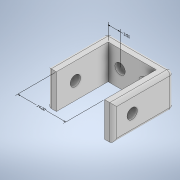
# Autodesk Inventor part: Part_B6
Saved by Autodesk Inventor 2022.6 (Build 266554010, 554A)
## iProperties
Created: 2025-05-30
Part Number: Part_B6
Material: Generic
Document SubType Name: Modeling
Designer: khinm
Density: 1 g/cm^3
Appearance: Default
Author: khinm
Autodesk Inventor part; units mm, degrees
ref_plane "YZ Plane" through (0, 0, 0) normal (1, 0, 0) x (0, 1, 0)
ref_plane "XZ Plane" through (0, 0, 0) normal (0, 1, 0) x (-1, 0, 0)
ref_plane "XY Plane" through (0, 0, 0) normal (0, 0, 1) x (1, 0, 0)
sketch "Sketch1" plane through (0, 0, 0) normal (0, 1, 0) x (-1, 0, 0)
  line L0 (7, -7.5) -> (-7, -7.5)
  line L1 (-7, -7.5) -> (-7, 7.5)
  line L2 (7, 7.5) -> (7, -7.5)
  line L3 (9.5, -10) -> (-9.5, -10)
  line L4 (9.5, 7.5) -> (9.5, -10)
  line L5 (7, 7.5) -> (9.5, 7.5)
  line L6 (-7, 7.5) -> (-9.5, 7.5)
  line L7 (-9.5, 7.5) -> (-9.5, -10)
  point P0 (0, 0)
  point P1 (0, -7.5)
  point P2 (7, 0)
  point P3 (9.5, 0)
  point P4 (0, -10)
  point P5 (8.25, 7.5)
  point P6 (-8.25, 7.5)
  dimension "d0" = 14
  dimension "d1" = 15
  dimension "d2" = 19
  dimension "d4" = 2.5
  constraints: 16 end point, 5 midpoint, 3 horizontal alignment, 2 horizontal, 2 parallel, 2 perpendicular, 2 point on line, 2 vertical alignment, 1 vertical
  measures "d0" distance of L0.start L0.end
  measures "d1" distance of L0.end L1.end
  measures "d2" distance of L3.start L3.end
  measures "d4" distance between parallel lines of L0 L3
extrude "Extrusion1" add sketch "Sketch1" along normal blind 10
sketch "Sketch2" plane through (-7, 0, -7.5) normal (0, 0, 1) x (1, 0, 0)
  point P0 (7, 0)
sketch "Sketch3" plane through (-7, 0, -7.5) normal (0, 0, 1) x (1, 0, 0)
  line L0 (0, 0) -> (14, 0) projected
  line L1 (14, 0) -> (14, 10) projected
  point P0 (7, 0)
  point P1 (10.5, 5)
  point P2 (3.5, 5)
  point P3 (7, 5)
  point P4 (7, 0)
  point P5 (14, 5)
  point P6 (7, 0)
  point P7 (7, 0)
  point P8 (14, 5)
  dimension "d7" = 7
  dimension "d8" = 3.5
  dimension "d9" = 3.5
  constraints: 5 midpoint, 2 horizontal alignment, 1 vertical alignment
  measures "d7" distance of point (3.5, 5) point (10.5, 5)
  measures "d8" horizontal distance of point (7, 0) point (3.5, 5)
  measures "d9" horizontal distance of point (10.5, 5) point (7, 0)
hole "Hole1" at (-3.5, 5, -7.5) at (3.5, 5, -7.5) direction (0, 0, -1) diameter 3 depth 2.5
sketch "Sketch4" plane through (9.5, 0, 7.5) normal (1, 0, 0) x (0, 0, -1)
  line L0 (17.5, 0) -> (17.5, 10) projected
  point P0 (7.5, 0)
  point P1 (5.5, 5)
  point P2 (15, 10)
  point P3 (17.5, 5)
  dimension "d21" = 9.5
  constraints: 1 horizontal alignment, 1 midpoint
  measures "d21" horizontal distance of point (15, 10) point (5.5, 5)
hole "Hole2" at (9.5, 5, 2) direction (-1, 0, 0) diameter 3 depth 19
fillet "Fillet1" radius 1 10 edges at (9.5, 10, -1.25) (9.5, 0, -1.25) (9.5, 5, 7.5) (9.5, 5, -10) (0, 10, -10) (0, 0, -10) (-9.5, 5, -10) (-9.5, 10, -1.25) (-9.5, 0, -1.25) (-9.5, 5, 7.5)
body "Solid1"
